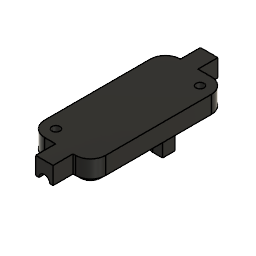
PE4 - PCB Case Lid (Autodesk Fusion 360 design; units mm, degrees)
Autodesk Fusion 360 part; units mm, degrees
sketch "Sketch1" plane through (0, 0, 0) normal (0, 0, 1) x (1, 0, 0)
  line L0 (6.2013, 11.75) -> (-6.2012, 11.75)
  line L1 (10.25, 10.25) -> (-10.25, -10.25) construction
  arc A0 (-6.2012, 11.75) -> (-11.75, 6.2013) centre (-6.2013, 6.2013) ccw
  line L2 (-11.75, 6.2013) -> (-11.75, -6.2013)
  arc A1 (-11.75, -6.2012) -> (-6.2012, -11.75) centre (-6.2013, -6.2013) ccw
  line L3 (-6.2012, -11.75) -> (6.2013, -11.75)
  arc A2 (11.75, 6.2012) -> (6.2013, 11.75) centre (6.2012, 6.2012) ccw
  arc A3 (6.2013, -11.75) -> (11.75, -6.2012) centre (6.2013, -6.2013) ccw
  line L4 (-10.25, 10.25) -> (10.25, -10.25) construction
  line L5 (11.75, -6.2012) -> (11.75, 6.2012)
  circle A4 centre (6.2012, 6.2012) radius 1.7
  circle A5 centre (-6.2013, -6.2013) radius 1.7
  line L6 (-6.2013, -6.2013) -> (-6.2013, -4) construction
  line L7 (-6.2013, -6.2013) -> (-4, -6.2013) construction
  line L8 (-4, -6.2013) -> (-4, -10.15)
  line L9 (-6.2013, -4) -> (-10.15, -4)
  line L10 (-4, -6.2013) -> (-4, -5)
  line L11 (-6.2013, -4) -> (-5, -4)
  arc A6 (-4, -5) -> (-5, -4) centre (-5, -5) ccw
  line L12 (6.2013, 4) -> (10.15, 4)
  line L13 (6.2013, 4) -> (5, 4)
  arc A7 (4, 5) -> (5, 4) centre (5, 5) ccw
  line L14 (4, 6.2013) -> (4, 5)
  line L15 (4, 6.2013) -> (4, 10.15)
  line L16 (10.15, -6.2012) -> (10.15, 6.2012)
  arc A8 (10.15, 6.2012) -> (6.2013, 10.15) centre (6.2012, 6.2012) ccw
  line L17 (6.2012, 10.15) -> (-6.2012, 10.15)
  arc A9 (-6.2012, 10.15) -> (-10.15, 6.2013) centre (-6.2013, 6.2013) ccw
  line L18 (-10.15, 6.2013) -> (-10.15, -6.2012)
  arc A10 (-10.15, -6.2012) -> (-6.2012, -10.15) centre (-6.2013, -6.2013) ccw
  line L19 (-6.2012, -10.15) -> (6.2013, -10.15)
  arc A11 (6.2013, -10.15) -> (10.15, -6.2013) centre (6.2013, -6.2013) ccw
  arc A12 (9.15, 6.2012) -> (6.2012, 9.15) centre (6.2012, 6.2012) ccw
  line L20 (6.2012, 9.15) -> (-6.2012, 9.15)
  arc A13 (-6.2012, 9.15) -> (-9.15, 6.2013) centre (-6.2013, 6.2013) ccw
  line L21 (-9.15, 6.2013) -> (-9.15, -6.2012)
  arc A14 (-9.15, -6.2012) -> (-6.2013, -9.15) centre (-6.2013, -6.2013) ccw
  line L22 (-6.2013, -9.15) -> (6.2013, -9.15)
  arc A15 (6.2013, -9.15) -> (9.15, -6.2013) centre (6.2013, -6.2013) ccw
  line L23 (9.15, -6.2013) -> (9.15, 6.2012)
  dimension "d2" = 20.5
  dimension "d3" = 20.5
  dimension "d8" = 3.4
  dimension "d9" = 3.4
  dimension "d13" = 1
  dimension "d26" = -1.6
  dimension "d27" = -2.6
  dimension "d89" = 5
  dimension "d90" = 9
  dimension "d91" = 9
  dimension "d92" = 6.75
  dimension "d93" = 1.2012
  dimension "d94" = 1
  dimension "d95" = 14.15
  dimension "d96" = 6.75
  dimension "d97" = 1.2012
  dimension "d98" = 14.15
  dimension "d99" = 2.2012
  dimension "d100" = 2.2012
  dimension "d101" = 2.2012
  dimension "d102" = 2.2012
  dimension "d103" = 135
  dimension "d104" = 5
  constraint coincident origin L1
  constraint coincident origin L4
  constraint vertical L6
  constraint perpendicular L6 L7
  constraint perpendicular L6 L9
  constraint perpendicular L7 L10
  constraint perpendicular L10 L11
  constraint tangent L10 A6
  constraint tangent L11 A6
  constraint vertical L15
  constraint horizontal L12
  constraint coincident L8.end L19
  constraint perpendicular L8 L19
  constraint coincident L9.end L18
  constraint perpendicular L9 L18
  constraint coincident L15.end L17
  constraint perpendicular L15 L17
  constraint coincident L12.end L16
  constraint perpendicular L12 L16
  constraint tangent A7 L14
  constraint tangent L13 A7
  constraint equal A6 A7
  constraint tangent A0 L2
  constraint tangent L0 A0
  constraint equal A0 A1
  constraint equal A0 A2
  constraint equal A0 A3
  constraint equal L10 L13
  constraint equal L10 L14
  constraint parallel L14 L15
  constraint parallel L12 L13
  constraint vertical L12.start L22.end
  constraint horizontal L14.start A12.start
  constraint midpoint origin L1
  constraint tangent L2 A1
  constraint equal L0 L2
  constraint equal L0 L18
  constraint equal L0 L21
  constraint equal L6 L7
  constraint equal L0 L23
  constraint equal L0 L16
  constraint equal L0 L5
  constraint tangent A1 L3
  constraint equal L0 L3
  constraint equal L0 L19
  constraint equal L0 L22
  constraint concentric A2 A4
  constraint concentric A1 A5
  constraint vertical L1.end L4.start
  constraint vertical L1.start L4.end
  constraint coincident A1.centre A5.centre
  measures "d2" distance of L1.start L4.start
  measures "d3" distance of L1.start L4.end
  measures "d8" diameter of A4
  measures "d9" diameter of A5
  measures "d13" radius of A6
  measures "d89" horizontal distance of origin A6.centre
  measures "d90" distance of A6.centre L13
  measures "d91" distance of A6.centre L14
  measures "d92" distance of L2 A6.centre
  measures "d93" distance of L6 A6.centre
  measures "d94" distance of L8 A6.centre
  measures "d95" distance of A6.centre L23
  measures "d96" distance of L3 A6.centre
  measures "d97" distance of L7 A6.centre
  measures "d98" distance of A6.centre L20
  measures "d99" distance of A0.centre L10
  measures "d100" distance of A3.centre L11
  measures "d101" distance of A2.centre L14
  measures "d102" distance of A2.centre L12
  measures "d103" angle of L1 L9
  measures "d104" vertical distance of origin A6.centre
sketch "Sketch2" plane through (0, 0, 0) normal (0, 0, 1) x (1, 0, 0)
  line L0 (-6.2013, -27.25) -> (6.2012, -27.25)
  arc A0 (6.2012, -27.25) -> (12.25, -21.2012) centre (6.2013, -21.2012) ccw
  line L1 (12.25, -21.2012) -> (12.25, 21.2013)
  arc A1 (12.25, 21.2013) -> (6.2013, 27.25) centre (6.2012, 21.2013) ccw
  line L2 (6.2013, 27.25) -> (-6.2012, 27.25)
  arc A2 (-6.2012, 27.25) -> (-12.25, 21.2013) centre (-6.2013, 21.2013) ccw
  line L3 (-12.25, 21.2013) -> (-12.25, -21.2012)
  arc A3 (-12.25, -21.2012) -> (-6.2013, -27.25) centre (-6.2013, -21.2012) ccw
  line L4 (-10.15, 21.2013) -> (-10.15, -21.2012)
  arc A4 (-10.15, -21.2012) -> (-6.2013, -25.15) centre (-6.2013, -21.2012) ccw
  line L5 (-6.2013, -25.15) -> (6.2013, -25.15)
  arc A5 (6.2013, -25.15) -> (10.15, -21.2012) centre (6.2013, -21.2012) ccw
  line L6 (10.15, -21.2012) -> (10.15, 17.8428)
  line L7 (2.8428, 25.15) -> (-6.2013, 25.15)
  arc A6 (-6.2013, 25.15) -> (-10.15, 21.2013) centre (-6.2013, 21.2013) ccw
  circle A7 centre (6.9428, 21.9428) radius 1.6
  circle A8 centre (-6.9428, -21.9428) radius 1.6
  line L8 (-6.2013, -25.15) -> (6.2012, -25.15)
  arc A9 (6.2012, -25.15) -> (10.15, -21.2012) centre (6.2013, -21.2012) ccw
  line L9 (10.15, -21.2012) -> (10.15, 21.2013)
  arc A10 (10.15, 21.2013) -> (6.2013, 25.15) centre (6.2012, 21.2013) ccw
  line L10 (6.2013, 25.15) -> (-6.2012, 25.15)
  arc A11 (-6.2012, 25.15) -> (-10.15, 21.2013) centre (-6.2013, 21.2013) ccw
  line L11 (-10.15, 21.2013) -> (-10.15, -21.2012)
  arc A12 (-10.15, -21.2012) -> (-6.2013, -25.15) centre (-6.2013, -21.2012) ccw
  line L12 (2.8428, 23.65) -> (-6.2013, 23.65)
  arc A13 (-6.2013, 23.65) -> (-8.65, 21.2013) centre (-6.2013, 21.2013) ccw
  line L13 (-8.65, 21.2013) -> (-8.65, -17.8428)
  line L14 (2.8428, 25.15) -> (2.8428, 23.65)
  line L15 (-8.65, -17.8428) -> (-10.15, -17.8428)
  line L16 (-2.8428, -23.65) -> (6.2013, -23.65)
  arc A14 (6.2013, -23.65) -> (8.65, -21.2012) centre (6.2013, -21.2012) ccw
  line L17 (8.65, -21.2012) -> (8.65, 17.8428)
  line L18 (-2.8428, -25.15) -> (-2.8428, -23.65)
  line L19 (10.15, 17.8428) -> (8.65, 17.8428)
  dimension "d62" = 3.2
  dimension "d63" = 3.2
  dimension "d71" = -2.1
  dimension "d105" = 8.65
  dimension "d106" = 17.8428
  dimension "d107" = 1.7072
  dimension "d108" = 15.5928
  dimension "d109" = 4.1
  dimension "d110" = 39.7857
  dimension "d111" = 6.0488
  dimension "d112" = 1.5
  dimension "d113" = 39.0441
  dimension "d114" = 2.4487
  dimension "d115" = 2.4488
  dimension "d116" = 5.8072
  dimension "d117" = 11.4928
  dimension "d118" = 14.8513
  dimension "d119" = 17.3
  dimension "d120" = 18.8
  dimension "d121" = 9.4072
  dimension "d122" = 5.8072
  dimension "d123" = 35.6857
  dimension "d124" = 7.3072
  dimension "d125" = 22.4
  dimension "d126" = 1.5
  constraint coincident L5 L18.start
  constraint perpendicular L7 L14
  constraint perpendicular L11 L15
  constraint coincident L4 L15.end
  constraint perpendicular L16 L18
  constraint perpendicular L17 L19
  constraint tangent A14 L17
  constraint tangent A13 L13
  constraint tangent L7 A11
  constraint tangent L3 A3
  constraint tangent L0 A3
  constraint tangent A2 L3
  constraint tangent L2 A2
  constraint tangent A1 L2
  constraint tangent L1 A1
  constraint tangent L0 A0
  constraint tangent A0 L1
  constraint concentric A6 A11
  constraint concentric A11 A13
  constraint concentric A3 A4
  constraint concentric A0 A5
  constraint coincident L4.start A11
  constraint perpendicular L13 L15
  constraint perpendicular L4 L15
  constraint equal A0 A3
  constraint equal A0 A2
  constraint equal A0 A1
  constraint equal L6 L13
  constraint equal L14 L15
  constraint midpoint A6 A11
  constraint midpoint L4 L11
  constraint parallel L0 L12
  constraint equal L7 L16
  measures "d62" diameter of A7
  measures "d63" diameter of A8
  measures "d105" distance of origin L13
  measures "d106" distance of origin L15
  measures "d107" distance of A8.centre L13
  measures "d108" distance of A7.centre L13
  measures "d109" distance of A8.centre L15
  measures "d110" distance of A7.centre L15
  measures "d111" radius of A2
  measures "d112" distance of L4.start L13
  measures "d113" distance of L1.end L15
  measures "d114" distance of L0.start L13
  measures "d115" distance of L2.end L13
  measures "d116" distance of L13 L18
  measures "d117" distance of L13 L14
  measures "d118" distance of A1.end L13
  measures "d119" distance of L13 L17
  measures "d120" distance of L9 L13
  measures "d121" distance of L0 L15
  measures "d122" distance of L15 L16
  measures "d123" distance of L15 L19
  measures "d124" distance of L18.start L15
  measures "d125" distance of L3 L6
  measures "d126" distance of A5 A14
extrude "Extrude5" add sketch "Sketch2" along normal blind 5 contours L0 A0 L1 A1 L2 A2 L3 A3 | L4 L7 A6 L10 A11 L11 L12 A13 L13 L14 L15 | L4 A4 L5 L8 L9 A10 L10 L11 A12 L12 A13 L13 L14 L15 L16 A14 L17 L18 L19 | L5 A5 L6 L8 A9 L9 L16 A14 L17 L18 L19 | A7 | A8
extrude "Extrude6" add sketch "Sketch2" against normal blind 2 contours L4 L7 A6 L10 A11 L11 L12 A13 L13 L14 L15 | L5 A5 L6 L8 A9 L9 L16 A14 L17 L18 L19
sketch "Sketch3" plane through (0, 0, 0) normal (0, 1, 0) x (1, 0, 0)
  line L0 (1.7, 3) -> (1.7, 0) construction
  line L1 (-0.45, 0) -> (-0.45, 2.15)
  line L2 (3.85, -0.0044) -> (3.85, 2.1456)
  line L3 (-0.45, 2.15) -> (3.85, 2.1456)
  arc A0 (1.7991, 2.1477) -> (1.6052, 2.1479) centre (1.7, 0) ccw
  arc A1 (-0.45, 0) -> (3.85, 0.0044) centre (1.7, 0) ccw
  line L4 (5.2, -5) -> (-1.8, -5)
  line L5 (-1.8, -5) -> (-1.8, 0)
  line L6 (5.2, 0) -> (5.2, -5)
  line L7 (5.2, -5) -> (0.1955, 2.1493) construction
  line L8 (-1.8, -5) -> (3.2024, 2.1463) construction
  line L9 (5.2, 0) -> (3.85, 0)
  line L10 (-0.45, 0) -> (-1.8, 0)
  point P0 (1.7, 0)
  dimension "d45" = 2.15
  dimension "d46" = 2.15
  dimension "d127" = 2.15
  dimension "d128" = 3.5
  dimension "d129" = 3.5
  dimension "d130" = 2.15
  dimension "d131" = 1.5045
  dimension "d132" = 1.5024
  dimension "d133" = 0.45
  dimension "d134" = 8
  constraint vertical L0
  constraint coincident L1.start A0
  constraint vertical L1
  constraint coincident L2.start A0
  constraint vertical L2
  constraint coincident L2 A1.end
  constraint coincident L3 A0.start
  constraint coincident L3 A0.end
  constraint concentric A0 A1
  constraint horizontal L4
  constraint perpendicular L4 L5
  constraint parallel L5 L6
  constraint coincident L7 P0
  constraint coincident L8 P0
  constraint coincident P0 L0.end
  constraint horizontal L9
  constraint coincident L3 L8.end
  constraint coincident L3 L7.end
  constraint coincident L2 L9.end
  constraint collinear L9 L10
  constraint horizontal origin L1.start
  constraint tangent L1 A1
  measures "d45" distance of L1.start L1.end
  measures "d46" distance of L2.start L2.end
  measures "d127" radius of A1
  measures "d128" distance of L0 L5
  measures "d129" distance of L0 L6
  measures "d130" distance of L0 L2
  measures "d131" distance of L0 L7.end
  measures "d132" distance of L0 L8.end
  measures "d133" distance of origin L1
  measures "d134" distance of L0.start L4
extrude "Extrude7" cut sketch "Sketch2" along normal blind 3 contours L4 A4 L5 L8 L9 A10 L10 L11 A12 L12 A13 L13 L14 L15 L16 A14 L17 L18 L19 | A7 | A8
extrude "Extrude8" cut sketch "Sketch3" against normal blind 31 contours L1 L2 L3 A0 A1
extrude "Extrude9" add sketch "Sketch3" against normal blind 8 from surface at -27.25 contours L2 A1 L4 L5 L6 L9 L10
sketch "Sketch4" plane through (0, 0, 0) normal (0, 1, 0) x (1, 0, 0)
  line L0 (6.2012, 4) -> (6.2, 4)
  line L1 (-6.2013, 0) -> (0.8, 0)
  line L2 (-4.85, 0) -> (-4.85, 2.15)
  line L3 (-4.85, 2.15) -> (-0.55, 2.1456)
  line L4 (-0.55, -0.0044) -> (-0.55, 2.1456)
  line L5 (-4.85, 0) -> (-2.7, 0) construction
  arc A0 (-4.85, 0) -> (-0.55, 0.0044) centre (-2.7, 0) ccw
  arc A1 (-2.6009, 2.1477) -> (-2.7948, 2.1479) centre (-2.7, 0) ccw
  line L6 (-6.2, -5) -> (0.8, -5)
  line L7 (0.8, -5) -> (0.8, 0)
  line L8 (-6.2, 0) -> (-6.2, -5)
  line L9 (-6.2, -5) -> (-1.1976, 2.1463) construction
  line L10 (0.8, -5) -> (-4.2045, 2.1493) construction
  line L11 (-4.85, 0) -> (-6.2013, 0)
  line L12 (-0.55, -0.0044) -> (0.8, 0)
  point P0 (-2.7, 0)
  dimension "d53" = 2.15
  dimension "d54" = 2.15
  dimension "d55" = 2.15
  dimension "d135" = 0.55
  dimension "d136" = 6.75
  dimension "d137" = 2.15
  dimension "d138" = 0.0044
  dimension "d139" = 1.35
  dimension "d140" = 4.9956
  dimension "d141" = 5.65
  dimension "d142" = 6.7513
  dimension "d143" = 4
  dimension "d144" = 5.6512
  constraint horizontal L1
  constraint horizontal L0
  constraint vertical L2
  constraint vertical L4
  constraint perpendicular L2 L5
  constraint coincident L3 A1.end
  constraint coincident L4 A0.end
  constraint coincident L3 A1.start
  constraint concentric A0 A1
  constraint horizontal L6
  constraint perpendicular L6 L7
  constraint parallel L7 L8
  constraint coincident L9 P0
  constraint coincident L10 P0
  constraint coincident P0 L5.end
  constraint perpendicular L8 L11
  constraint coincident L3 L9.end
  constraint coincident L3 L10.end
  constraint coincident L1 L8.start
  constraint tangent L2 A0
  constraint coincident L4.start A0
  constraint equal A0 A1
  constraint coincident origin L1
  measures "d53" distance of L2.start L2.end
  measures "d54" distance of L3.end L4.start
  measures "d55" distance of L2.start P0
  measures "d135" distance of origin L4
  measures "d136" distance of L0.end L4
  measures "d137" radius of A0
  measures "d138" distance of L4.start L5
  measures "d139" distance of L4 L7
  measures "d140" distance of L4.start L6
  measures "d141" distance of L4 L8
  measures "d142" distance of L0.start L4
  measures "d143" distance of L0 L11
  measures "d144" distance of L1.start L4
extrude "Extrude10" add sketch "Sketch4" along normal blind 8 from surface at 27.25 contours L1 A0 L6 L7 L8 L11 L12
extrude "Extrude11" cut sketch "Sketch4" along normal blind 61 contours L1 L2 L3 L4 A0 A1 | L1 L4 A0
extrude "Extrude12" cut sketch "Sketch2" along normal blind 20 contours A7 | A8
extrude "Extrude13" add 1 faces at (-4.3101, 7.137, 5) along direction (0, 0, 1) blind 2
sketch "Sketch5" plane through (0, 0, 3) normal (0, 0, -1) x (1, 0, 0)
  circle A0 centre (6.9428, -21.9428) radius 1.6
  circle A1 centre (-6.9428, 21.9428) radius 1.6
  arc A2 (-6.2013, 25.15) -> (-10.15, 21.2012) centre (-6.2013, 21.2012) ccw
  line L0 (-10.15, 21.2012) -> (-10.15, 17.8428)
  line L1 (2.8428, -25.15) -> (6.2013, -25.15)
  arc A3 (6.2013, -25.15) -> (10.15, -21.2013) centre (6.2012, -21.2013) ccw
  line L2 (10.15, -21.2013) -> (10.15, -17.8428)
  line L3 (9.15, -17.8428) -> (-9.15, -17.8428)
  line L4 (-9.15, -17.8428) -> (-9.15, 17.8428)
  line L5 (-9.15, 17.8428) -> (9.15, 17.8428)
  line L6 (9.15, 17.8428) -> (9.15, -17.8428)
  line L7 (-10.15, 17.8428) -> (-8.65, 17.8428)
  line L8 (-8.65, 17.8428) -> (-8.65, -21.2013)
  arc A4 (-8.65, -21.2013) -> (-6.2013, -23.65) centre (-6.2013, -21.2013) ccw
  line L9 (-6.2013, -23.65) -> (2.8428, -23.65)
  line L10 (2.8428, -23.65) -> (2.8428, -25.15)
  line L11 (10.15, -17.8428) -> (8.65, -17.8428)
  line L12 (8.65, -17.8428) -> (8.65, 21.2012)
  arc A5 (8.65, 21.2012) -> (6.2013, 23.65) centre (6.2013, 21.2012) ccw
  line L13 (6.2013, 23.65) -> (-2.8428, 23.65)
  line L14 (-2.8428, 23.65) -> (-2.8428, 25.15)
  line L15 (-2.8428, 25.15) -> (-6.2013, 25.15)
  dimension "d145" = 1
  dimension "d146" = 18.3
  constraint horizontal L3
  constraint vertical L4
  constraint horizontal L5
  constraint vertical L6
  constraint coincident L3.start L11
  constraint coincident L4.end L7
  measures "d145" distance of L0.end L4
  measures "d146" distance of L4 L6
extrude "Extrude14" cut sketch "Sketch5" against normal blind 2 contours L3 L4 L5 L7 L8 | L3 L5 L8 L12 | L3 L5 L6 L11 L12
sketch "Sketch6" plane through (0, 0, 5) normal (0, 0, -1) x (1, 0, 0)
  line L0 (9.15, 17.8428) -> (-9.15, 17.8428)
  line L1 (-9.15, 17.8428) -> (-9.15, -17.8428)
  line L2 (-9.15, -17.8428) -> (9.15, -17.8428)
  line L3 (9.15, -17.8428) -> (9.15, 17.8428)
  line L4 (6.2012, -6.2012) -> (6.2012, -3.7012) construction
  line L5 (6.2012, -3.7012) -> (9.15, -3.7012)
  line L6 (9.15, -8.7012) -> (6.2012, -8.7012)
  arc A0 (6.2012, -3.7012) -> (6.2012, -8.7012) centre (6.2012, -6.2012) ccw
  line L7 (-6.2013, 3.7013) -> (-9.15, 3.7013)
  line L8 (-9.15, 8.7013) -> (-6.2013, 8.7013)
  arc A1 (-6.2013, 3.7013) -> (-6.2013, 8.7013) centre (-6.2013, 6.2013) ccw
  line L9 (-9.15, 3.7013) -> (-10.15, 3.7013)
  line L10 (-10.15, 3.7013) -> (-10.15, 8.7013)
  line L11 (-10.15, 8.7013) -> (-9.15, 8.7013)
  line L12 (9.15, -8.7012) -> (10.15, -8.7012)
  line L13 (10.15, -8.7012) -> (10.15, -3.7012)
  line L14 (10.15, -3.7012) -> (9.15, -3.7012)
  dimension "d75" = 5
  dimension "d76" = 5
  dimension "d79" = 1
  dimension "d80" = 5
  dimension "d81" = 1
  dimension "d82" = 5
  dimension "d147" = 15.3512
  dimension "d148" = 21.5441
  dimension "d149" = 14.1416
  constraint coincident L4.start A0.centre
  constraint parallel L5 L6
  constraint parallel L7 L8
  constraint horizontal L9
  constraint vertical L10
  constraint horizontal L11
  constraint horizontal L12
  constraint vertical L13
  constraint horizontal L14
  constraint tangent L7 A1
  constraint tangent L8 A1
  constraint tangent L6 A0
  constraint tangent L5 A0
  constraint coincident L1 L7.end
  constraint coincident L1 L8.start
  constraint coincident L3 L5.end
  constraint coincident L3 L6.start
  constraint equal L5 L7
  measures "d75" diameter of A1
  measures "d76" diameter of A0
  measures "d79" distance of L7.end L9.end
  measures "d80" distance of L7.end L8.start
  measures "d81" distance of L6.start L12.end
  measures "d82" distance of L6.start L5.end
  measures "d147" distance of L1 L4
  measures "d148" distance of L2 L7
  measures "d149" distance of L2 L5
extrude "Extrude15" add sketch "Sketch6" along normal blind 12.45 contours L3 L12 L13 L14 | L3 L5 L6 A0 | L1 L7 L8 A1 | L1 L9 L10 L11
extrude "Extrude16" add 1 faces at (-2.0372, -23.65, 0.4401) along direction (0, 1, 0) blind 2
extrude "Extrude17" add 1 faces at (1.7037, 23.65, 0.4415) along direction (0, -1, 0) blind 2
equation "d45 = ( 4.3 / 2 ) * 1 mm"
equation "d46 = ( 4.3 / 2 ) * 1 mm"
equation "d53 = ( 4.3 / 2 ) * 1 mm"
equation "d54 = ( 4.3 / 2 ) * 1 mm"
equation "d55 = ( 4.3 / 2 ) * 1 mm"
equation "d77 = 5.00 mm + 7.45 mm"
